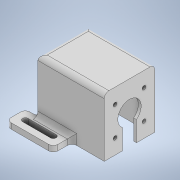
# Autodesk Inventor part: NEMA17_Shroud
Saved by Autodesk Inventor 2021 (Build 250183000, 183)
## iProperties
Created: 2021-10-06
Part Number: NEMA17_Shroud
Material: Generic
Document SubType Name: Modeling
Designer: Jorian Brusind
Density: 1 g/cm^3
Appearance: Default
Author: Jorian Brusind
Autodesk Inventor part; units mm, degrees
ref_plane "YZ Plane" through (0, 0, 0) normal (1, 0, 0) x (0, 1, 0)
ref_plane "XZ Plane" through (0, 0, 0) normal (0, 1, 0) x (-1, 0, 0)
ref_plane "XY Plane" through (0, 0, 0) normal (0, 0, 1) x (1, 0, 0)
sketch "Sketch1" plane through (0, 0, 0) normal (0, 1, 0) x (-1, 0, 0)
  line L0 (0, 0) -> (65, 0)
  line L1 (65, 0) -> (65, -48)
  line L2 (65, -48) -> (0, -48)
  line L3 (0, -51) -> (68, -51)
  line L4 (68, -51) -> (68, 3)
  line L5 (68, 3) -> (0, 3)
  line L6 (0, 3) -> (0, 0)
  line L7 (0, -48) -> (0, -51)
  dimension "d0" = 65
  dimension "d1" = 48
  dimension "d2" = 3
  dimension "d96" = 65
  constraints: 16 end point, 3 equal length, 2 perpendicular, 1 horizontal, 1 vertical, 2 other
  measures "d0" distance of L1.end L2.end
  measures "d1" distance of L0.end L1.end
  measures "d2" distance between parallel lines of L1 L4
  measures "d96" distance between parallel lines of L6 L1
extrude "Extrusion1" add sketch "Sketch1" along normal blind 60
sketch "Sketch2" plane through (0, 60, 0) normal (0, 1, 0) x (1, 0, 0)
  line L0 (-68, 51) -> (-68, -3) projected
  line L1 (0, 48) -> (0, 51) projected
  line L2 (-68, -3) -> (0, -3)
  line L3 (0, -3) -> (0, 51)
  line L4 (0, 51) -> (-68, 51)
  line L5 (-68, 51) -> (-68, -3)
  point P0 (0, 0)
  constraints: 8 end point, 2 parallel, 1 horizontal, 1 perpendicular
extrude "Extrusion2" add sketch "Sketch2" along normal blind 3
ref_plane "Work Plane1" through (0, -5, 0) normal (0, -1, 0) x (1, 0, 0)
ref_plane "Work Plane2" through (5, 60, 0) normal (1, 0, 0) x (0, 0, -1)
fillet "Fillet11" radius 5 3 edges at (-34, 63, 3) (-34, 63, -51) (-68, 63, -24)
sketch "Sketch5" plane through (0, 0, 0) normal (0, -1, 0) x (1, 0, 0)
  line L0 (-68, 3) -> (0, 3) projected
  line L1 (0, -51) -> (-68, -51) projected
  line L2 (-31.5, 3) -> (-81.5, 3)
  line L3 (-81.5, 3) -> (-81.5, 23)
  line L4 (-81.5, 23) -> (-31.5, 23)
  line L5 (-31.5, 23) -> (-31.5, 3)
  line L6 (0, -51) -> (-68, -51) projected
  line L7 (-31.5, -51) -> (-81.5, -51)
  line L8 (-81.5, -51) -> (-81.5, -71)
  line L9 (-81.5, -71) -> (-31.5, -71)
  line L10 (-31.5, -71) -> (-31.5, -51)
  line L11 (-81.5, 13) -> (-71.5, 13)
  line L12 (-81.5, -61) -> (-71.5, -61)
  line L13 (-71.5, 13) -> (-41.5, 13) construction
  line L14 (-71.5, 10) -> (-41.5, 10)
  line L15 (-41.5, 16) -> (-71.5, 16)
  arc A0 (-71.5, 16) -> (-71.5, 10) centre (-71.5, 13) ccw
  arc A1 (-41.5, 10) -> (-41.5, 16) centre (-41.5, 13) ccw
  line L16 (-71.5, -61) -> (-41.5, -61) construction
  line L17 (-71.5, -64) -> (-41.5, -64)
  line L18 (-41.5, -58) -> (-71.5, -58)
  arc A2 (-71.5, -58) -> (-71.5, -64) centre (-71.5, -61) ccw
  arc A3 (-41.5, -64) -> (-41.5, -58) centre (-41.5, -61) ccw
  line L19 (-71.5, -61) -> (-41.5, -61) construction
  point P0 (-63, 3)
  point P1 (-63, -51)
  point P2 (-56.5, 13)
  point P3 (-56.5, -61)
  point P4 (-63, 3)
  dimension "d132" = 50
  dimension "d133" = 20
  dimension "d134" = 50
  dimension "d135" = 20
  dimension "d136" = 10
  dimension "d137" = 10
  dimension "d138" = 30
  dimension "d139" = 6
  dimension "d140" = 30
  dimension "d141" = 0
  dimension "d142" = 6
  constraints: 38 end point, 8 point on circle, 8 tangent, 7 parallel, 6 horizontal, 4 centre point, 4 midpoint, 2 perpendicular, 2 point on line, 1 collinear
  measures "d132" distance of L3.end L4.end
  measures "d133" distance of L2.end L3.end
  measures "d134" distance of L9.end L8.end
  measures "d135" distance of L8.end L7.end
  measures "d136" distance of L11.start L11.end
  measures "d137" distance of L12.start L12.end
  measures "d138" distance of L11.end L13.end
  measures "d139" diameter of A1
  measures "d140" distance of L12.end L16.end
  measures "d141" distance between parallel lines of L16 L19
  measures "d142" diameter of A3
sketch "Sketch6" plane through (0, 60, 0) normal (1, 0, 0) x (0, 0, -1)
  line L0 (2, -60) -> (-3, -60) projected
  line L1 (-3, -60) -> (51, -60)
  line L2 (51, -60) -> (51, 3)
  line L3 (51, 3) -> (-3, 3)
  line L4 (-3, 3) -> (-3, -60)
  dimension "d109" = 54
  dimension "d110" = 63
  constraints: 8 end point, 2 parallel, 1 horizontal, 1 perpendicular
  measures "d109" distance of L3.end L2.end
  measures "d110" distance of L2.end L1.end
extrude "Extrusion6" add sketch "Sketch6" along normal blind 3
fillet "Fillet19" radius 5 2 edges at (1.5, 63, -51) (1.5, 63, 3)
sketch "Sketch10" plane through (3, 60, 0) normal (1, 0, 0) x (0, 0, -1)
  circle A0 centre (8.5, -13) radius 2
  arc A1 (2, 3) -> (-3, -2) centre (2, -2) ccw projected
  arc A2 (51, -2) -> (46, 3) centre (46, -2) ccw projected
  line L0 (2, 3) -> (46, 3)
  line L1 (-3, -60) -> (-3, -2) projected
  line L2 (-3, -2) -> (-3, -54)
  circle A3 centre (39.5, -13) radius 2
  circle A4 centre (8.5, -44) radius 2
  circle A5 centre (39.5, -44) radius 2
  point P0 (0, -60)
  dimension "d112" = 4
  dimension "d115" = 31
  dimension "d118" = 31
  dimension "d121" = 11.5
  dimension "d122" = 16
  constraints: 4 centre point, 4 end point, 2 horizontal, 2 vertical, 1 tangent, 6 other
  measures "d112" diameter of A0
  measures "d115" distance of A0.centre A3.centre
  measures "d118" distance of A0.centre A4.centre
  measures "d121" distance from line of L1 A0.centre
  measures "d122" distance from line of L0 A0.centre
extrude "Extrusion10" cut sketch "Sketch10" against normal blind 3
sketch "Sketch11" plane through (3, 60, 0) normal (1, 0, 0) x (0, 0, -1)
  circle A0 centre (39.5, -44) radius 2 projected
  circle A1 centre (8.5, -13) radius 2 projected
  line L0 (39.5, -44) -> (8.5, -13)
  circle A2 centre (8.5, -44) radius 2 projected
  circle A3 centre (39.5, -13) radius 2 projected
  line L1 (8.5, -44) -> (39.5, -13)
  circle A4 centre (24, -28.5) radius 12.5
  line L2 (24, -28.5) -> (24, -60)
  line L3 (0, -60) -> (48, -60) projected
  line L4 (24, -28.5) -> (55.5, -28.5) construction
  line L5 (24, -60) -> (31.5, -60)
  line L6 (31.5, -60) -> (16.5, -60)
  line L7 (16.5, -60) -> (16.5, -38.5)
  line L8 (16.5, -38.5) -> (31.5, -38.5)
  line L9 (31.5, -38.5) -> (31.5, -60)
  dimension "d125" = 25
  dimension "d126" = 90
  dimension "d127" = 7.5
  dimension "d128" = 15
  dimension "d129" = 21.5
  constraints: 18 end point, 2 horizontal, 2 midpoint, 2 parallel, 2 perpendicular, 1 centre point, 1 point on line
  measures "d125" diameter of A4
  measures "d126" angle of L2 L4
  measures "d127" distance of L2.end L5.end
  measures "d128" distance of L7.end L8.end
  measures "d129" distance of L6.end L7.end
extrude "Extrusion11" cut sketch "Sketch11" against normal blind 3 contours A4 L8 L2 L0 | L0 L1 A4 | L1 A4 L0 | L2 L8 A4 L1 | L0 A4 L1 | L9 L3 L2 A4 | A4 L2 L8 | L2 A4 L8 | L2 L3 L7 A4
extrude "Extrusion12" add sketch "Sketch5" against normal blind 6
fillet "Fillet20" radius 5 8 edges at (-81.5, 3, -71) (-31.5, 3, -71) (-81.5, 3, -51) (-81.5, 3, 3) (-81.5, 3, 23) (-31.5, 3, 23) (-31.5, 3, -51) (-31.5, 3, 3)
fillet "Fillet21" radius 5 2 edges at (-68, 3, -51) (-68, 3, 3)
fillet "Fillet22" radius 5 2 edges at (-47.25, 6, -51) (-47.25, 6, 3)
body "Solid1"
